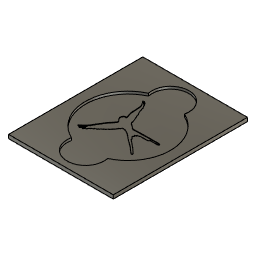
Wingspan - Food Token Lid (Autodesk Fusion 360 design; units mm, degrees)
Autodesk Fusion 360 part; units mm, degrees
(part 1 of 2)
sketch "Skizze1" plane through (0, 0, 0) normal (0, 0, 1) x (1, 0, 0)
  line L0 (0, 0) -> (85, 0)
  line L1 (85, 0) -> (85, 109)
  line L2 (85, 109) -> (0, 109)
  line L3 (0, 109) -> (0, 0)
  line L4 (0, 0) -> (7, 0)
  line L5 (7, 0) -> (7, 7)
  line L6 (7, 7) -> (0, 7)
  line L7 (0, 7) -> (0, 0)
  line L8 (85, 0) -> (78, 0)
  line L9 (78, 0) -> (78, 7)
  line L10 (78, 7) -> (85, 7)
  line L11 (85, 7) -> (85, 0)
  line L12 (85, 109) -> (78, 109)
  line L13 (78, 109) -> (78, 102)
  line L14 (78, 102) -> (85, 102)
  line L15 (85, 102) -> (85, 109)
  line L16 (0, 109) -> (7, 109)
  line L17 (7, 109) -> (7, 102)
  line L18 (7, 102) -> (0, 102)
  line L19 (0, 102) -> (0, 109)
  circle A0 centre (3.5, 3.5) radius 2.65
  circle A1 centre (81.5, 3.5) radius 2.65
  circle A2 centre (81.5, 105.5) radius 2.65
  circle A3 centre (3.5, 105.5) radius 2.65
  dimension "d1" = 85
  dimension "d2" = 109
  dimension "d3" = 7
  dimension "d4" = 7
  dimension "d5" = 7
  dimension "d6" = 7
  dimension "d7" = 7
  dimension "d8" = 7
  dimension "d9" = 7
  dimension "d10" = 7
  dimension "d11" = 5.3
  dimension "d12" = 5.3
  dimension "d13" = 5.3
  dimension "d14" = 5.3
  dimension "d15" = 3.5
  dimension "d16" = 3.5
  dimension "d17" = 3.5
  dimension "d18" = 3.5
  dimension "d19" = 3.5
  dimension "d20" = 3.5
  dimension "d21" = 3.5
  dimension "d22" = 3.5
  constraint horizontal L0
  constraint vertical L1
  constraint horizontal L2
  constraint vertical L3
  constraint coincident L0.start L3.end
  constraint horizontal L4
  constraint vertical L5
  constraint horizontal L6
  constraint vertical L7
  constraint horizontal L8
  constraint vertical L9
  constraint horizontal L10
  constraint vertical L11
  constraint horizontal L12
  constraint vertical L13
  constraint horizontal L14
  constraint vertical L15
  constraint horizontal L16
  constraint vertical L17
  constraint horizontal L18
  constraint vertical L19
  measures "d1" distance of L0.start L0.end
  measures "d2" distance of L0.start L2.end
  measures "d3" distance of L0.start L4.end
  measures "d4" distance of L0.start L6.end
  measures "d5" distance of L0.end L8.end
  measures "d6" distance of L0.end L10.end
  measures "d7" distance of L1.end L12.end
  measures "d8" distance of L1.end L14.end
  measures "d9" distance of L2.end L16.end
  measures "d10" distance of L2.end L18.end
  measures "d11" diameter of A0
  measures "d12" diameter of A1
  measures "d13" diameter of A2
  measures "d14" diameter of A3
  measures "d15" distance of L19 A3.centre
  measures "d16" distance of L16 A3.centre
  measures "d17" distance of L2 A2.centre
  measures "d18" distance of L1 A2.centre
  measures "d19" distance of L1 A1.centre
  measures "d20" distance of L0 A1.centre
  measures "d21" distance of L0 A0.centre
  measures "d22" distance of L5 A0.centre
extrude "Extrusion3" add sketch "Skizze1" along normal blind 3 contours L0 L3 L4 L5 L6 L7 | L0 L1 L2 L3 L5 L6 L9 L10 L13 L14 L17 L18 | L0 L1 L8 L9 L10 L11 | L2 L3 L16 L17 L18 L19 | L1 L2 L12 L13 L14 L15 | A0 | A1 | A2 | A3
extrude "Extrusion4" cut sketch "Skizze1" along normal blind 1.2 contours A0 | A1 | A2 | A3
sketch "Skizze3" plane through (0, 0, 3) normal (0, 0, 1) x (-1, 0, 0)
  line L0 (0, -109) -> (0, 0)
  line L1 (0, 0) -> (-85, 0)
  line L2 (-85, 0) -> (-85, -109)
  line L3 (-85, -109) -> (0, -109)
  circle A0 centre (-42.5, -54.5) radius 34.5
  circle A1 centre (-42.5, -89) radius 15
  circle A2 centre (-42.5, -20) radius 15
  dimension "d39" = 69
  dimension "d40" = 42.5
  dimension "d50" = 30
  dimension "d51" = 30
  dimension "d52" = 20
  dimension "d53" = 20
  constraint coincident A0 A1.centre
  constraint coincident A0 A2.centre
  measures "d39" diameter of A0
  measures "d40" distance of L2 A0.centre
  measures "d50" diameter of A1
  measures "d51" diameter of A2
  measures "d52" distance of L1 A2.centre
  measures "d53" distance of L3 A1.centre
extrude "Extrusion7" cut sketch "Skizze3" against normal blind 2 contours A0 A1 A2 | A0 A2 | A0 A2 | A0 A1 | A0 A1
sketch "Skizze5" plane through (0, 0, 1) normal (0, 0, 1) x (-1, 0, 0)
  arc A0 (-27.8587, -23.2609) -> (-57.1413, -23.2609) centre (-42.5, -20) ccw
  arc A1 (-57.1413, -23.2609) -> (-57.1413, -85.7391) centre (-42.5, -54.5) ccw
  arc A2 (-57.1413, -85.7391) -> (-27.8587, -85.7391) centre (-42.5, -89) ccw
  arc A3 (-27.8587, -85.7391) -> (-27.8587, -23.2609) centre (-42.5, -54.5) ccw
  spline S0 degree 3 poles (-66.4769, -55.696) (-66.34, -55.5333) (-66.0829, -55.391) (-65.7535, -55.2957) knots 0 0 0 0 1 1 1 1
  spline S1 degree 3 poles (-65.7535, -55.2957) (-65.527, -55.2301) (-64.4525, -55.1908) (-60.9377, -55.1195) knots 0 0 0 0 1 1 1 1
  line L0 (-60.9377, -55.1195) -> (-59.6311, -55.0929)
  line L1 (-59.6311, -55.0929) -> (-59.5794, -54.9682)
  spline S2 degree 3 poles (-59.5794, -54.9682) (-59.551, -54.8996) (-59.4198, -54.7368) (-59.2878, -54.6065) knots 0 0 0 0 1 1 1 1
  spline S3 degree 3 poles (-59.2878, -54.6065) (-59.1032, -54.4242) (-58.9697, -54.341) (-58.7092, -54.2459) knots 0 0 0 0 1 1 1 1
  line L2 (-58.7092, -54.2459) -> (-58.3706, -54.1223)
  line L3 (-58.3706, -54.1223) -> (-56.297, -54.1159)
  spline S4 degree 3 poles (-56.297, -54.1159) (-55.1565, -54.1124) (-53.92, -54.1227) (-53.5492, -54.1387) knots 0 0 0 0 1 1 1 1
  line L4 (-53.5492, -54.1387) -> (-52.875, -54.1678)
  line L5 (-52.875, -54.1678) -> (-52.7061, -53.9931)
  spline S5 degree 3 poles (-52.7061, -53.9931) (-52.3675, -53.6427) (-52.283, -53.6204) (-51.3104, -53.6252) knots 0 0 0 0 1 1 1 1
  line L6 (-51.3104, -53.6252) -> (-50.4482, -53.6294)
  line L7 (-50.4482, -53.6294) -> (-50.6724, -53.5227)
  spline S6 degree 3 poles (-50.6724, -53.5227) (-51.098, -53.3202) (-51.2581, -53.0214) (-51.0466, -52.8244) knots 0 0 0 0 1 1 1 1
  spline S7 degree 3 poles (-51.0466, -52.8244) (-50.8983, -52.6862) (-50.6376, -52.6297) (-50.0763, -52.6141) knots 0 0 0 0 1 1 1 1
  spline S8 degree 3 poles (-50.0763, -52.6141) (-49.8005, -52.6065) (-49.5647, -52.5989) (-49.5522, -52.5973) knots 0 0 0 0 1 1 1 1
  spline S9 degree 3 poles (-49.5522, -52.5973) (-49.5396, -52.5958) (-49.6513, -52.5267) (-49.8002, -52.4438) knots 0 0 0 0 1 1 1 1
  spline S10 degree 3 poles (-49.8002, -52.4438) (-50.1699, -52.2381) (-50.2586, -52.1091) (-50.2586, -51.7767) knots 0 0 0 0 1 1 1 1
  spline S11 degree 3 poles (-50.2586, -51.7767) (-50.2586, -51.5758) (-50.2364, -51.4865) (-50.1674, -51.4091) knots 0 0 0 0 1 1 1 1
  spline S12 degree 3 poles (-50.1674, -51.4091) (-50.0289, -51.2538) (-49.7965, -51.172) (-49.592, -51.2065) knots 0 0 0 0 1 1 1 1
  spline S13 degree 3 poles (-49.592, -51.2065) (-49.3888, -51.2409) (-49.3721, -51.2026) (-49.5262, -51.0565) knots 0 0 0 0 1 1 1 1
  spline S14 degree 3 poles (-49.5262, -51.0565) (-49.5863, -50.9995) (-49.662, -50.8491) (-49.6945, -50.7222) knots 0 0 0 0 1 1 1 1
  spline S15 degree 3 poles (-49.6945, -50.7222) (-49.7368, -50.5571) (-49.7967, -50.4568) (-49.9045, -50.3699) knots 0 0 0 0 1 1 1 1
  spline S16 degree 3 poles (-49.9045, -50.3699) (-50.9398, -49.5366) (-51.2613, -49.1022) (-51.2611, -48.537) knots 0 0 0 0 1 1 1 1
  line L8 (-51.2611, -48.537) -> (-51.261, -48.2382)
  line L9 (-51.261, -48.2382) -> (-51.6839, -47.9217)
  spline S17 degree 3 poles (-51.6839, -47.9217) (-52.6699, -47.184) (-53.8348, -46.2825) (-54.2425, -45.9418) knots 0 0 0 0 1 1 1 1
  spline S18 degree 3 poles (-54.2425, -45.9418) (-54.4075, -45.8039) (-54.6394, -45.6132) (-54.7578, -45.5181) knots 0 0 0 0 1 1 1 1
  spline S19 degree 3 poles (-54.7578, -45.5181) (-54.8763, -45.423) (-54.9993, -45.3205) (-55.0313, -45.2903) knots 0 0 0 0 1 1 1 1
  spline S20 degree 3 poles (-55.0313, -45.2903) (-55.0633, -45.2601) (-55.2433, -45.1022) (-55.4312, -44.9393) knots 0 0 0 0 1 1 1 1
  spline S21 degree 3 poles (-55.4312, -44.9393) (-55.6192, -44.7764) (-55.7832, -44.632) (-55.7957, -44.6185) knots 0 0 0 0 1 1 1 1
  spline S22 degree 3 poles (-55.7957, -44.6185) (-55.8083, -44.605) (-56.0339, -44.4246) (-56.297, -44.2177) knots 0 0 0 0 1 1 1 1
  spline S23 degree 3 poles (-56.297, -44.2177) (-57.2107, -43.4994) (-57.9229, -42.9318) (-58.0098, -42.8527) knots 0 0 0 0 1 1 1 1
  spline S24 degree 3 poles (-58.0098, -42.8527) (-58.0579, -42.8089) (-58.156, -42.7275) (-58.2279, -42.6719) knots 0 0 0 0 1 1 1 1
  spline S25 degree 3 poles (-58.2279, -42.6719) (-58.4581, -42.4936) (-58.8082, -42.168) (-59.5801, -41.4142) knots 0 0 0 0 1 1 1 1
  spline S26 degree 3 poles (-59.5801, -41.4142) (-59.9946, -41.0094) (-60.4764, -40.5551) (-60.6506, -40.4047) knots 0 0 0 0 1 1 1 1
  spline S27 degree 3 poles (-60.6506, -40.4047) (-61.2019, -39.9288) (-61.5559, -39.5916) (-61.7517, -39.3554) knots 0 0 0 0 1 1 1 1
  spline S28 degree 3 poles (-61.7517, -39.3554) (-62.1736, -38.8466) (-62.3005, -38.3445) (-62.0559, -38.1521) knots 0 0 0 0 1 1 1 1
  spline S29 degree 3 poles (-62.0559, -38.1521) (-61.9898, -38.1002) (-61.8911, -38.0577) (-61.8365, -38.0577) knots 0 0 0 0 1 1 1 1
  spline S30 degree 3 poles (-61.8365, -38.0577) (-61.5957, -38.0577) (-61.0744, -38.3909) (-60.2553, -39.0684) knots 0 0 0 0 1 1 1 1
  spline S31 degree 3 poles (-60.2553, -39.0684) (-59.6798, -39.5445) (-57.8513, -41.1473) (-57.4333, -41.5422) knots 0 0 0 0 1 1 1 1
  spline S32 degree 3 poles (-57.4333, -41.5422) (-56.8243, -42.1176) (-56.0099, -42.7891) (-55.4142, -43.2072) knots 0 0 0 0 1 1 1 1
  spline S33 degree 3 poles (-55.4142, -43.2072) (-55.3608, -43.2446) (-55.1224, -43.425) (-54.8842, -43.6081) knots 0 0 0 0 1 1 1 1
  spline S34 degree 3 poles (-54.8842, -43.6081) (-54.6461, -43.7911) (-54.2975, -44.0573) (-54.1095, -44.1995) knots 0 0 0 0 1 1 1 1
  spline S35 degree 3 poles (-54.1095, -44.1995) (-53.9215, -44.3418) (-53.7574, -44.47) (-53.7449, -44.4844) knots 0 0 0 0 1 1 1 1
  spline S36 degree 3 poles (-53.7449, -44.4844) (-53.6626, -44.579) (-52.9747, -45.0648) (-52.1726, -45.5948) knots 0 0 0 0 1 1 1 1
  spline S37 degree 3 poles (-52.1726, -45.5948) (-51.947, -45.7439) (-51.5599, -46.0213) (-51.3124, -46.2115) knots 0 0 0 0 1 1 1 1
  spline S38 degree 3 poles (-51.3124, -46.2115) (-51.0649, -46.4016) (-50.6119, -46.7417) (-50.3058, -46.9672) knots 0 0 0 0 1 1 1 1
  spline S39 degree 3 poles (-50.3058, -46.9672) (-49.9997, -47.1928) (-49.6491, -47.4594) (-49.5267, -47.5597) knots 0 0 0 0 1 1 1 1
  spline S40 degree 3 poles (-49.5267, -47.5597) (-49.4043, -47.66) (-49.2625, -47.7758) (-49.2117, -47.8172) knots 0 0 0 0 1 1 1 1
  spline S41 degree 3 poles (-49.2117, -47.8172) (-48.9391, -48.0387) (-48.6357, -48.303) (-48.4128, -48.5129) knots 0 0 0 0 1 1 1 1
  spline S42 degree 3 poles (-48.4128, -48.5129) (-47.9347, -48.9631) (-47.2927, -49.4869) (-46.5933, -49.9973) knots 0 0 0 0 1 1 1 1
  spline S43 degree 3 poles (-46.5933, -49.9973) (-46.2067, -50.2794) (-45.8395, -50.5574) (-45.7774, -50.615) knots 0 0 0 0 1 1 1 1
  spline S44 degree 3 poles (-45.7774, -50.615) (-45.7153, -50.6726) (-45.552, -50.7628) (-45.4146, -50.8154) knots 0 0 0 0 1 1 1 1
  spline S45 degree 3 poles (-45.4146, -50.8154) (-45.2771, -50.868) (-45.034, -51.0024) (-44.8742, -51.114) knots 0 0 0 0 1 1 1 1
  spline S46 degree 3 poles (-44.8742, -51.114) (-44.7145, -51.2257) (-44.4968, -51.3657) (-44.3905, -51.4251) knots 0 0 0 0 1 1 1 1
  spline S47 degree 3 poles (-44.3905, -51.4251) (-44.2843, -51.4846) (-44.0127, -51.6369) (-43.7871, -51.7636) knots 0 0 0 0 1 1 1 1
  spline S48 degree 3 poles (-43.7871, -51.7636) (-43.2146, -52.0851) (-42.9986, -52.1776) (-42.3972, -52.3586) knots 0 0 0 0 1 1 1 1
  spline S49 degree 3 poles (-42.3972, -52.3586) (-42.3094, -52.385) (-42.0736, -52.4366) (-41.8731, -52.4733) knots 0 0 0 0 1 1 1 1
  spline S50 degree 3 poles (-41.8731, -52.4733) (-40.6244, -52.7018) (-40.1267, -52.7538) (-40.0297, -52.666) knots 0 0 0 0 1 1 1 1
  spline S51 degree 3 poles (-40.0297, -52.666) (-39.9907, -52.6308) (-39.9025, -52.5805) (-39.8336, -52.5543) knots 0 0 0 0 1 1 1 1
  spline S52 degree 3 poles (-39.8336, -52.5543) (-39.7276, -52.514) (-39.7083, -52.4802) (-39.7079, -52.3346) knots 0 0 0 0 1 1 1 1
  spline S53 degree 3 poles (-39.7079, -52.3346) (-39.7074, -52.1249) (-39.5052, -51.7553) (-39.2857, -51.5625) knots 0 0 0 0 1 1 1 1
  spline S54 degree 3 poles (-39.2857, -51.5625) (-39.1997, -51.487) (-38.9728, -51.3245) (-38.7815, -51.2015) knots 0 0 0 0 1 1 1 1
  spline S55 degree 3 poles (-38.7815, -51.2015) (-38.4753, -51.0044) (-38.4336, -50.9613) (-38.433, -50.8403) knots 0 0 0 0 1 1 1 1
  spline S56 degree 3 poles (-38.433, -50.8403) (-38.4319, -50.6375) (-38.2757, -50.3745) (-37.9723, -50.065) knots 0 0 0 0 1 1 1 1
  spline S57 degree 3 poles (-37.9723, -50.065) (-37.7651, -49.8536) (-37.7031, -49.759) (-37.7031, -49.6542) knots 0 0 0 0 1 1 1 1
  spline S58 degree 3 poles (-37.7031, -49.6542) (-37.7031, -49.3952) (-37.486, -49.0956) (-36.7303, -48.3117) knots 0 0 0 0 1 1 1 1
  spline S59 degree 3 poles (-36.7303, -48.3117) (-36.605, -48.1817) (-36.5214, -48.0471) (-36.5021, -47.9442) knots 0 0 0 0 1 1 1 1
  spline S60 degree 3 poles (-36.5021, -47.9442) (-36.4668, -47.7556) (-36.3035, -47.5861) (-35.8816, -47.2996) knots 0 0 0 0 1 1 1 1
  spline S61 degree 3 poles (-35.8816, -47.2996) (-35.6517, -47.1435) (-35.5802, -47.0676) (-35.5572, -46.9547) knots 0 0 0 0 1 1 1 1
  spline S62 degree 3 poles (-35.5572, -46.9547) (-35.5232, -46.7888) (-35.4056, -46.595) (-35.2684, -46.4787) knots 0 0 0 0 1 1 1 1
  spline S63 degree 3 poles (-35.2684, -46.4787) (-35.1092, -46.3439) (-34.6422, -46.1241) (-34.5148, -46.1241) knots 0 0 0 0 1 1 1 1
  spline S64 degree 3 poles (-34.5148, -46.1241) (-34.3507, -46.1241) (-34.2851, -46.0455) (-34.2851, -45.8486) knots 0 0 0 0 1 1 1 1
  spline S65 degree 3 poles (-34.2851, -45.8486) (-34.2851, -45.6239) (-34.1771, -45.4147) (-33.9272, -45.1554) knots 0 0 0 0 1 1 1 1
  spline S66 degree 3 poles (-33.9272, -45.1554) (-33.7648, -44.9869) (-33.6355, -44.9073) (-33.3475, -44.7986) knots 0 0 0 0 1 1 1 1
  line L10 (-33.3475, -44.7986) -> (-32.9769, -44.6588)
  line L11 (-32.9769, -44.6588) -> (-32.845, -44.3828)
  spline S67 degree 3 poles (-32.845, -44.3828) (-32.7703, -44.2264) (-32.631, -44.0346) (-32.5238, -43.9402) knots 0 0 0 0 1 1 1 1
  spline S68 degree 3 poles (-32.5238, -43.9402) (-32.2976, -43.7411) (-31.8763, -43.5265) (-31.7117, -43.5265) knots 0 0 0 0 1 1 1 1
  spline S69 degree 3 poles (-31.7117, -43.5265) (-31.6466, -43.5265) (-31.5858, -43.5008) (-31.5764, -43.4695) knots 0 0 0 0 1 1 1 1
  spline S70 degree 3 poles (-31.5764, -43.4695) (-31.4482, -43.041) (-31.3897, -42.8961) (-31.2943, -42.771) knots 0 0 0 0 1 1 1 1
  spline S71 degree 3 poles (-31.2943, -42.771) (-31.1591, -42.5937) (-31.0965, -42.563) (-30.7991, -42.5279) knots 0 0 0 0 1 1 1 1
  spline S72 degree 3 poles (-30.7991, -42.5279) (-30.6026, -42.5047) (-30.5683, -42.4855) (-30.5484, -42.3871) knots 0 0 0 0 1 1 1 1
  spline S73 degree 3 poles (-30.5484, -42.3871) (-30.5357, -42.3245) (-30.468, -42.1707) (-30.3978, -42.0453) knots 0 0 0 0 1 1 1 1
  spline S74 degree 3 poles (-30.3978, -42.0453) (-30.1637, -41.6269) (-29.6643, -41.3954) (-29.1645, -41.4736) knots 0 0 0 0 1 1 1 1
  line L12 (-29.1645, -41.4736) -> (-28.943, -41.5083)
  line L13 (-28.943, -41.5083) -> (-28.8747, -41.3439)
  spline S75 degree 3 poles (-28.8747, -41.3439) (-28.5136, -40.4738) (-28.2322, -40.1996) (-27.7003, -40.1996) knots 0 0 0 0 1 1 1 1
  spline S76 degree 3 poles (-27.7003, -40.1996) (-27.5176, -40.1996) (-27.4862, -40.1846) (-27.4379, -40.0743) knots 0 0 0 0 1 1 1 1
  spline S77 degree 3 poles (-27.4379, -40.0743) (-27.3216, -39.8085) (-26.9953, -39.3413) (-26.8574, -39.2431) knots 0 0 0 0 1 1 1 1
  spline S78 degree 3 poles (-26.8574, -39.2431) (-26.7338, -39.1551) (-26.6213, -39.1237) (-26.3759, -39.1088) knots 0 0 0 0 1 1 1 1
  spline S79 degree 3 poles (-26.3759, -39.1088) (-26.3496, -39.1072) (-26.3014, -39.029) (-26.2687, -38.935) knots 0 0 0 0 1 1 1 1
  spline S80 degree 3 poles (-26.2687, -38.935) (-26.0867, -38.4114) (-25.7297, -37.7861) (-25.5326, -37.6458) knots 0 0 0 0 1 1 1 1
  spline S81 degree 3 poles (-25.5326, -37.6458) (-25.3618, -37.5242) (-25.2466, -37.5595) (-25.1499, -37.7631) knots 0 0 0 0 1 1 1 1
  spline S82 degree 3 poles (-25.1499, -37.7631) (-25.1087, -37.8499) (-25.0606, -37.9209) (-25.043, -37.9208) knots 0 0 0 0 1 1 1 1
  spline S83 degree 3 poles (-25.043, -37.9208) (-25.0254, -37.9207) (-24.9723, -37.8266) (-24.925, -37.7116) knots 0 0 0 0 1 1 1 1
  spline S84 degree 3 poles (-24.925, -37.7116) (-24.6067, -36.9378) (-23.588, -35.957) (-23.457, -36.2982) knots 0 0 0 0 1 1 1 1
  spline S85 degree 3 poles (-23.457, -36.2982) (-23.4357, -36.3538) (-23.5936, -36.8575) (-23.7586, -37.2601) knots 0 0 0 0 1 1 1 1
  spline S86 degree 3 poles (-23.7586, -37.2601) (-23.8232, -37.4177) (-23.8414, -37.4655) (-24.0021, -37.8982) knots 0 0 0 0 1 1 1 1
  spline S87 degree 3 poles (-24.0021, -37.8982) (-24.1251, -38.2292) (-24.1962, -38.5134) (-24.1561, -38.5134) knots 0 0 0 0 1 1 1 1
  spline S88 degree 3 poles (-24.1561, -38.5134) (-24.1433, -38.5134) (-24.0038, -38.334) (-23.846, -38.1146) knots 0 0 0 0 1 1 1 1
  spline S89 degree 3 poles (-23.846, -38.1146) (-23.5032, -37.6383) (-22.5753, -36.5191) (-22.2944, -36.2433) knots 0 0 0 0 1 1 1 1
  spline S90 degree 3 poles (-22.2944, -36.2433) (-21.9373, -35.8927) (-21.479, -35.6325) (-21.479, -35.7804) knots 0 0 0 0 1 1 1 1
  spline S91 degree 3 poles (-21.479, -35.7804) (-21.479, -35.8063) (-21.679, -36.0602) (-21.9234, -36.3448) knots 0 0 0 0 1 1 1 1
  spline S92 degree 3 poles (-21.9234, -36.3448) (-22.4445, -36.9516) (-22.5938, -37.14) (-22.7745, -37.4189) knots 0 0 0 0 1 1 1 1
  spline S93 degree 3 poles (-22.7745, -37.4189) (-23.0018, -37.7697) (-23.2586, -38.253) (-23.2318, -38.2797) knots 0 0 0 0 1 1 1 1
  spline S94 degree 3 poles (-23.2318, -38.2797) (-23.2178, -38.2937) (-22.8638, -37.9588) (-22.4452, -37.5353) knots 0 0 0 0 1 1 1 1
  spline S95 degree 3 poles (-22.4452, -37.5353) (-21.8538, -36.937) (-21.579, -36.6961) (-21.2126, -36.4545) knots 0 0 0 0 1 1 1 1
  spline S96 degree 3 poles (-21.2126, -36.4545) (-20.948, -36.28) (-20.6914, -36.1436) (-20.6278, -36.1436) knots 0 0 0 0 1 1 1 1
  spline S97 degree 3 poles (-20.6278, -36.1436) (-20.4556, -36.1436) (-20.5179, -36.2337) (-20.8387, -36.4486) knots 0 0 0 0 1 1 1 1
  spline S98 degree 3 poles (-20.8387, -36.4486) (-21.1871, -36.6821) (-21.5614, -37.004) (-22.0473, -37.4881) knots 0 0 0 0 1 1 1 1
  spline S99 degree 3 poles (-22.0473, -37.4881) (-22.7212, -38.1595) (-23.0746, -38.62) (-23.6485, -39.5745) knots 0 0 0 0 1 1 1 1
  spline S100 degree 3 poles (-23.6485, -39.5745) (-23.9868, -40.137) (-24.0053, -40.2286) (-23.7285, -39.97) knots 0 0 0 0 1 1 1 1
  spline S101 degree 3 poles (-23.7285, -39.97) (-23.5024, -39.7589) (-23.346, -39.6291) (-22.6639, -39.0863) knots 0 0 0 0 1 1 1 1
  spline S102 degree 3 poles (-22.6639, -39.0863) (-22.4509, -38.9168) (-22.1433, -38.6518) (-21.9803, -38.4974) knots 0 0 0 0 1 1 1 1
  spline S103 degree 3 poles (-21.9803, -38.4974) (-21.3863, -37.9344) (-20.9782, -37.5964) (-20.5158, -37.2843) knots 0 0 0 0 1 1 1 1
  spline S104 degree 3 poles (-20.5158, -37.2843) (-20.256, -37.109) (-19.9438, -36.8934) (-19.822, -36.8052) knots 0 0 0 0 1 1 1 1
  spline S105 degree 3 poles (-19.822, -36.8052) (-19.6003, -36.6447) (-19.458, -36.6054) (-19.4057, -36.6901) knots 0 0 0 0 1 1 1 1
  spline S106 degree 3 poles (-19.4057, -36.6901) (-19.3728, -36.7433) (-19.4722, -36.8384) (-19.9779, -37.2374) knots 0 0 0 0 1 1 1 1
  spline S107 degree 3 poles (-19.9779, -37.2374) (-20.988, -38.0342) (-21.6759, -38.6504) (-22.5637, -39.5537) knots 0 0 0 0 1 1 1 1
  spline S108 degree 3 poles (-22.5637, -39.5537) (-23.0976, -40.0969) (-23.6206, -40.6605) (-23.7258, -40.8061) knots 0 0 0 0 1 1 1 1
  spline S109 degree 3 poles (-23.7258, -40.8061) (-23.8311, -40.9516) (-24.0012, -41.1807) (-24.1038, -41.3152) knots 0 0 0 0 1 1 1 1
  spline S110 degree 3 poles (-24.1038, -41.3152) (-24.5569, -41.9085) (-25.3728, -43.1972) (-25.706, -43.8455) knots 0 0 0 0 1 1 1 1
  spline S111 degree 3 poles (-25.706, -43.8455) (-26.1808, -44.7695) (-26.3303, -45.0267) (-26.7764, -45.6872) knots 0 0 0 0 1 1 1 1
  spline S112 degree 3 poles (-26.7764, -45.6872) (-27.6231, -46.9408) (-28.2239, -47.8712) (-28.2239, -47.9288) knots 0 0 0 0 1 1 1 1
  spline S113 degree 3 poles (-28.2239, -47.9288) (-28.2239, -47.9399) (-28.272, -48.0254) (-28.3309, -48.1189) knots 0 0 0 0 1 1 1 1
  spline S114 degree 3 poles (-28.3309, -48.1189) (-28.3897, -48.2124) (-28.51, -48.4222) (-28.5981, -48.5851) knots 0 0 0 0 1 1 1 1
  spline S115 degree 3 poles (-28.5981, -48.5851) (-28.6863, -48.748) (-28.8057, -48.9634) (-28.8636, -49.0636) knots 0 0 0 0 1 1 1 1
  spline S116 degree 3 poles (-28.8636, -49.0636) (-28.9215, -49.1639) (-29.0219, -49.3382) (-29.0867, -49.451) knots 0 0 0 0 1 1 1 1
  spline S117 degree 3 poles (-29.0867, -49.451) (-29.1515, -49.5638) (-29.2761, -49.7575) (-29.3636, -49.8815) knots 0 0 0 0 1 1 1 1
  spline S118 degree 3 poles (-29.3636, -49.8815) (-29.6443, -50.2791) (-31.007, -51.9697) (-31.865, -52.9847) knots 0 0 0 0 1 1 1 1
  spline S119 degree 3 poles (-31.865, -52.9847) (-32.0366, -53.1877) (-32.8129, -54.2308) (-32.9999, -54.5096) knots 0 0 0 0 1 1 1 1
  spline S120 degree 3 poles (-32.9999, -54.5096) (-33.4602, -55.196) (-33.5128, -55.3056) (-33.5059, -55.5654) knots 0 0 0 0 1 1 1 1
  spline S121 degree 3 poles (-33.5059, -55.5654) (-33.4939, -56.0167) (-33.2865, -56.3551) (-32.7659, -56.7729) knots 0 0 0 0 1 1 1 1
  spline S122 degree 3 poles (-32.7659, -56.7729) (-31.8731, -57.4895) (-31.4629, -58.0581) (-31.2493, -58.8755) knots 0 0 0 0 1 1 1 1
  spline S123 degree 3 poles (-31.2493, -58.8755) (-31.1724, -59.1695) (-31.1648, -60.1497) (-31.238, -60.3295) knots 0 0 0 0 1 1 1 1
  spline S124 degree 3 poles (-31.238, -60.3295) (-31.5742, -61.1551) (-31.915, -61.6094) (-32.3837, -61.8568) knots 0 0 0 0 1 1 1 1
  spline S125 degree 3 poles (-32.3837, -61.8568) (-32.6571, -62.0011) (-33.3043, -62.0003) (-33.5987, -61.8554) knots 0 0 0 0 1 1 1 1
  spline S126 degree 3 poles (-33.5987, -61.8554) (-34.0207, -61.6476) (-34.0797, -61.7272) (-33.9054, -62.2693) knots 0 0 0 0 1 1 1 1
  spline S127 degree 3 poles (-33.9054, -62.2693) (-33.831, -62.5007) (-33.7563, -62.7208) (-33.7395, -62.7584) knots 0 0 0 0 1 1 1 1
  spline S128 degree 3 poles (-33.7395, -62.7584) (-33.6155, -63.0353) (-32.7433, -65.8249) (-32.6423, -66.2675) knots 0 0 0 0 1 1 1 1
  spline S129 degree 3 poles (-32.6423, -66.2675) (-32.6108, -66.4054) (-32.5574, -66.6062) (-32.5236, -66.7137) knots 0 0 0 0 1 1 1 1
  spline S130 degree 3 poles (-32.5236, -66.7137) (-32.357, -67.2428) (-32.3173, -67.6943) (-32.3001, -69.2526) knots 0 0 0 0 1 1 1 1
  spline S131 degree 3 poles (-32.3001, -69.2526) (-32.2908, -70.1048) (-32.2639, -70.9456) (-32.2404, -71.1211) knots 0 0 0 0 1 1 1 1
  spline S132 degree 3 poles (-32.2404, -71.1211) (-32.1632, -71.6977) (-32.1063, -72.2947) (-32.0557, -73.0579) knots 0 0 0 0 1 1 1 1
  spline S133 degree 3 poles (-32.0557, -73.0579) (-31.9862, -74.1079) (-31.8116, -75.4244) (-31.6841, -75.8607) knots 0 0 0 0 1 1 1 1
  spline S134 degree 3 poles (-31.6841, -75.8607) (-31.4966, -76.5023) (-31.3516, -76.7732) (-30.7569, -77.5925) knots 0 0 0 0 1 1 1 1
  spline S135 degree 3 poles (-30.7569, -77.5925) (-29.8366, -78.8604) (-29.6535, -79.1189) (-29.4185, -79.4825) knots 0 0 0 0 1 1 1 1
  spline S136 degree 3 poles (-29.4185, -79.4825) (-28.9782, -80.1639) (-28.9489, -80.2297) (-29.0663, -80.2748) knots 0 0 0 0 1 1 1 1
  spline S137 degree 3 poles (-29.0663, -80.2748) (-29.1292, -80.2989) (-29.4694, -80.0351) (-29.9784, -79.5675) knots 0 0 0 0 1 1 1 1
  spline S138 degree 3 poles (-29.9784, -79.5675) (-30.0787, -79.4754) (-30.2149, -79.3577) (-30.281, -79.3059) knots 0 0 0 0 1 1 1 1
  spline S139 degree 3 poles (-30.281, -79.3059) (-30.3471, -79.2541) (-30.5108, -79.0767) (-30.6446, -78.9118) knots 0 0 0 0 1 1 1 1
  spline S140 degree 3 poles (-30.6446, -78.9118) (-30.7784, -78.7468) (-30.8953, -78.6339) (-30.9042, -78.6608) knots 0 0 0 0 1 1 1 1
  spline S141 degree 3 poles (-30.9042, -78.6608) (-30.947, -78.7891) (-30.1803, -79.9438) (-29.8888, -80.1902) knots 0 0 0 0 1 1 1 1
  spline S142 degree 3 poles (-29.8888, -80.1902) (-29.8591, -80.2152) (-29.7982, -80.2921) (-29.7533, -80.3611) knots 0 0 0 0 1 1 1 1
  spline S143 degree 3 poles (-29.7533, -80.3611) (-29.6732, -80.4841) (-29.6735, -80.4864) (-29.7691, -80.4864) knots 0 0 0 0 1 1 1 1
  spline S144 degree 3 poles (-29.7691, -80.4864) (-29.8519, -80.4864) (-30.0572, -80.3286) (-30.3633, -80.0298) knots 0 0 0 0 1 1 1 1
  spline S145 degree 3 poles (-30.3633, -80.0298) (-30.7613, -79.6411) (-31.2149, -78.9699) (-31.4855, -78.369) knots 0 0 0 0 1 1 1 1
  spline S146 degree 3 poles (-31.4855, -78.369) (-31.6468, -78.0109) (-31.7338, -77.8939) (-31.7325, -78.0368) knots 0 0 0 0 1 1 1 1
  spline S147 degree 3 poles (-31.7325, -78.0368) (-31.7316, -78.1411) (-31.4114, -79.0011) (-31.2979, -79.2041) knots 0 0 0 0 1 1 1 1
  spline S148 degree 3 poles (-31.2979, -79.2041) (-31.1648, -79.4424) (-31.157, -79.5293) (-31.269, -79.5293) knots 0 0 0 0 1 1 1 1
  spline S149 degree 3 poles (-31.269, -79.5293) (-31.4614, -79.5293) (-32.1902, -78.2413) (-32.4424, -77.4558) knots 0 0 0 0 1 1 1 1
  spline S150 degree 3 poles (-32.4424, -77.4558) (-32.5482, -77.126) (-32.61, -77.0823) (-32.6358, -77.319) knots 0 0 0 0 1 1 1 1
  spline S151 degree 3 poles (-32.6358, -77.319) (-32.656, -77.5053) (-32.7468, -77.5978) (-32.8212, -77.5081) knots 0 0 0 0 1 1 1 1
  spline S152 degree 3 poles (-32.8212, -77.5081) (-32.8699, -77.4494) (-33.2525, -76.4156) (-33.3129, -76.1797) knots 0 0 0 0 1 1 1 1
  spline S153 degree 3 poles (-33.3129, -76.1797) (-33.3583, -76.0024) (-33.4868, -75.7915) (-33.5646, -75.7668) knots 0 0 0 0 1 1 1 1
  spline S154 degree 3 poles (-33.5646, -75.7668) (-33.6451, -75.7412) (-33.9953, -75.2362) (-34.0955, -75.0011) knots 0 0 0 0 1 1 1 1
  spline S155 degree 3 poles (-34.0955, -75.0011) (-34.1261, -74.9293) (-34.164, -74.6422) (-34.1796, -74.363) knots 0 0 0 0 1 1 1 1
  spline S156 degree 3 poles (-34.1796, -74.363) (-34.2081, -73.8564) (-34.2085, -73.8551) (-34.3812, -73.6578) knots 0 0 0 0 1 1 1 1
  spline S157 degree 3 poles (-34.3812, -73.6578) (-34.6559, -73.344) (-34.742, -73.12) (-34.7815, -72.6162) knots 0 0 0 0 1 1 1 1
  spline S158 degree 3 poles (-34.7815, -72.6162) (-34.8145, -72.1951) (-34.8288, -72.1481) (-35.0294, -71.8037) knots 0 0 0 0 1 1 1 1
  spline S159 degree 3 poles (-35.0294, -71.8037) (-35.1724, -71.5582) (-35.2774, -71.2996) (-35.3489, -71.0169) knots 0 0 0 0 1 1 1 1
  spline S160 degree 3 poles (-35.3489, -71.0169) (-35.4089, -70.7795) (-35.4962, -70.5512) (-35.5489, -70.4938) knots 0 0 0 0 1 1 1 1
  spline S161 degree 3 poles (-35.5489, -70.4938) (-35.7137, -70.3142) (-35.9158, -69.9436) (-35.9908, -69.6833) knots 0 0 0 0 1 1 1 1
  spline S162 degree 3 poles (-35.9908, -69.6833) (-36.0475, -69.4864) (-36.1068, -69.3943) (-36.2588, -69.2673) knots 0 0 0 0 1 1 1 1
  spline S163 degree 3 poles (-36.2588, -69.2673) (-36.5572, -69.0178) (-36.7051, -68.6949) (-36.7351, -68.2272) knots 0 0 0 0 1 1 1 1
  spline S164 degree 3 poles (-36.7351, -68.2272) (-36.7546, -67.9231) (-36.7839, -67.8017) (-36.8716, -67.6624) knots 0 0 0 0 1 1 1 1
  spline S165 degree 3 poles (-36.8716, -67.6624) (-37.0892, -67.3168) (-37.3841, -66.6596) (-37.3841, -66.5202) knots 0 0 0 0 1 1 1 1
  spline S166 degree 3 poles (-37.3841, -66.5202) (-37.3841, -66.4224) (-37.4554, -66.2813) (-37.616, -66.0612) knots 0 0 0 0 1 1 1 1
  spline S167 degree 3 poles (-37.616, -66.0612) (-37.9268, -65.6353) (-38.0221, -65.4065) (-38.0221, -65.0859) knots 0 0 0 0 1 1 1 1
  spline S168 degree 3 poles (-38.0221, -65.0859) (-38.0221, -64.8763) (-38.0416, -64.8058) (-38.1185, -64.7365) knots 0 0 0 0 1 1 1 1
  spline S169 degree 3 poles (-38.1185, -64.7365) (-38.2777, -64.593) (-38.4922, -64.0881) (-38.4972, -63.8448) knots 0 0 0 0 1 1 1 1
  spline S170 degree 3 poles (-38.4972, -63.8448) (-38.5012, -63.6545) (-38.5254, -63.6025) (-38.6896, -63.432) knots 0 0 0 0 1 1 1 1
  spline S171 degree 3 poles (-38.6896, -63.432) (-39.0848, -63.0217) (-39.2763, -62.5524) (-39.1944, -62.1947) knots 0 0 0 0 1 1 1 1
  spline S172 degree 3 poles (-39.1944, -62.1947) (-39.151, -62.0051) (-39.1565, -61.9799) (-39.271, -61.8438) knots 0 0 0 0 1 1 1 1
  spline S173 degree 3 poles (-39.271, -61.8438) (-39.5749, -61.4827) (-39.7064, -61.0329) (-39.6201, -60.6505) knots 0 0 0 0 1 1 1 1
  spline S174 degree 3 poles (-39.6201, -60.6505) (-39.5743, -60.4475) (-39.5791, -60.423) (-39.698, -60.259) knots 0 0 0 0 1 1 1 1
  spline S175 degree 3 poles (-39.698, -60.259) (-39.7677, -60.1627) (-39.8611, -60.0038) (-39.9055, -59.9059) knots 0 0 0 0 1 1 1 1
  spline S176 degree 3 poles (-39.9055, -59.9059) (-39.9612, -59.783) (-40.081, -59.6605) (-40.2916, -59.511) knots 0 0 0 0 1 1 1 1
  spline S177 degree 3 poles (-40.2916, -59.511) (-41.0321, -58.9854) (-43.0088, -57.5318) (-43.198, -57.3738) knots 0 0 0 0 1 1 1 1
  spline S178 degree 3 poles (-43.198, -57.3738) (-43.2684, -57.3149) (-43.4092, -57.1928) (-43.511, -57.1023) knots 0 0 0 0 1 1 1 1
  spline S179 degree 3 poles (-43.511, -57.1023) (-43.6127, -57.0118) (-43.8981, -56.7804) (-44.1451, -56.5881) knots 0 0 0 0 1 1 1 1
  line L14 (-44.1451, -56.5881) -> (-44.5942, -56.2385)
  line L15 (-44.5942, -56.2385) -> (-44.9199, -56.2631)
  spline S180 degree 3 poles (-44.9199, -56.2631) (-45.3621, -56.2965) (-48.1545, -56.3703) (-50.213, -56.403) knots 0 0 0 0 1 1 1 1
  spline S181 degree 3 poles (-50.213, -56.403) (-51.1404, -56.4178) (-52.3914, -56.4601) (-52.9929, -56.497) knots 0 0 0 0 1 1 1 1
  spline S182 degree 3 poles (-52.9929, -56.497) (-53.8407, -56.5491) (-54.9325, -56.5612) (-57.8465, -56.5509) knots 0 0 0 0 1 1 1 1
  spline S183 degree 3 poles (-57.8465, -56.5509) (-62.7312, -56.5337) (-63.9953, -56.543) (-64.6564, -56.6012) knots 0 0 0 0 1 1 1 1
  spline S184 degree 3 poles (-64.6564, -56.6012) (-65.0967, -56.64) (-65.283, -56.6361) (-65.6363, -56.5807) knots 0 0 0 0 1 1 1 1
  spline S185 degree 3 poles (-65.6363, -56.5807) (-66.1781, -56.4958) (-66.2885, -56.4524) (-66.4601, -56.257) knots 0 0 0 0 1 1 1 1
  spline S186 degree 3 poles (-66.4601, -56.257) (-66.6314, -56.0618) (-66.6367, -55.8859) (-66.4769, -55.696) knots 0 0 0 0 1 1 1 1
  spline S187 degree 3 poles (-24.967, -41.4757) (-24.9553, -41.4757) (-24.9212, -41.4295) (-24.8912, -41.3731) knots 0 0 0 0 1 1 1 1
  spline S188 degree 3 poles (-24.8912, -41.3731) (-24.8416, -41.2802) (-24.8436, -41.2764) (-24.9124, -41.3331) knots 0 0 0 0 1 1 1 1
  spline S189 degree 3 poles (-24.9124, -41.3331) (-24.9829, -41.3914) (-25.0153, -41.4757) (-24.967, -41.4757) knots 0 0 0 0 1 1 1 1
extrude "Extrusion8" cut sketch "Skizze5" against normal blind 0.4 contours S0 S1 L0 L1 S2 S3 L2 L3 S4 L4 L5 S5 L6 L7 S6 S7 S8 S9 S10 S11 S12 S13 S14 S15 S16 L8 L9 S17 S18 S19 S20 S21 S22 S23 S24 S25 S26 S27 S28 S29 S30 S31 S32 S33 S34 S35 S36 S37 S38 S39 S40 S41 S42 S43 S44 S45 S46 S47 S48 S49 S50 S51 S52 S53 S54 S55 S56 S57 S58 S59 S60 S61 S62 S63 S64 S65 S66 L10 L11 S67 S68 S69 S70 S71 S72 S73 S74 L12 L13 S75 S76 S77 S78 S79 S80 S81 S82 S83 S84 S85 S86 S87 S88 S89 S90 S91 S92 S93 S94 S95 S96 S97 S98 S99 S100 S101 S102 S103 S104 S105 S106 S107 S108 S109 S110 S111 S112 S113 S114 S115 S116 S117 S118 S119 S120 S121 S122 S123 S124 S125 S126 S127 S128 S129 S130 S131 S132 S133 S134 S135 S136 S137 S138 S139 S140 S141 S142 S143 S144 S145 S146 S147 S148 S149 S150 S151 S152 S153 S154 S155 S156 S157 S158 S159 S160 S161 S162 S163 S164 S165 S166 S167 S168 S169 S170 S171 S172 S173 S174 S175 S176 S177 S178 S179 L14 L15 S180 S181 S182 S183 S184 S185 S186
extrude "Extrusion5" [suppressed]
sketch "Skizze4" plane through (0, 0, 1) normal (0, 0, 1) x (-1, 0, 0)
  arc A0 (-27.8484, -22.7143) -> (-57.1516, -22.7143) centre (-42.5, -19.5) ccw
  arc A1 (-57.1516, -22.7143) -> (-57.1516, -86.2857) centre (-42.5, -54.5) ccw
  arc A2 (-57.1516, -86.2857) -> (-27.8484, -86.2857) centre (-42.5, -89.5) ccw
  arc A3 (-27.8484, -86.2857) -> (-27.8484, -22.7143) centre (-42.5, -54.5) ccw
  spline S0 degree 3 poles (-70.5128, -55.4557) (-70.3599, -55.2739) (-70.0727, -55.115) (-69.7047, -55.0084) knots 0 0 0 0 1 1 1 1
  spline S1 degree 3 poles (-69.7047, -55.0084) (-69.4517, -54.9352) (-68.2513, -54.8913) (-64.325, -54.8116) knots 0 0 0 0 1 1 1 1
  line L0 (-64.325, -54.8116) -> (-62.8653, -54.782)
  line L1 (-62.8653, -54.782) -> (-62.8076, -54.6426)
  spline S2 degree 3 poles (-62.8076, -54.6426) (-62.7759, -54.566) (-62.6293, -54.3841) (-62.4818, -54.2385) knots 0 0 0 0 1 1 1 1
  spline S3 degree 3 poles (-62.4818, -54.2385) (-62.2756, -54.0349) (-62.1265, -53.9419) (-61.8355, -53.8357) knots 0 0 0 0 1 1 1 1
  line L2 (-61.8355, -53.8357) -> (-61.4572, -53.6976)
  line L3 (-61.4572, -53.6976) -> (-59.1408, -53.6905)
  spline S4 degree 3 poles (-59.1408, -53.6905) (-57.8667, -53.6866) (-56.4854, -53.6981) (-56.0712, -53.716) knots 0 0 0 0 1 1 1 1
  line L4 (-56.0712, -53.716) -> (-55.318, -53.7485)
  line L5 (-55.318, -53.7485) -> (-55.1293, -53.5533)
  spline S5 degree 3 poles (-55.1293, -53.5533) (-54.751, -53.1618) (-54.6567, -53.137) (-53.5702, -53.1423) knots 0 0 0 0 1 1 1 1
  line L6 (-53.5702, -53.1423) -> (-52.607, -53.1471)
  line L7 (-52.607, -53.1471) -> (-52.8575, -53.0279)
  spline S6 degree 3 poles (-52.8575, -53.0279) (-53.3329, -52.8016) (-53.5118, -52.4679) (-53.2755, -52.2478) knots 0 0 0 0 1 1 1 1
  spline S7 degree 3 poles (-53.2755, -52.2478) (-53.1098, -52.0933) (-52.8185, -52.0302) (-52.1915, -52.0129) knots 0 0 0 0 1 1 1 1
  spline S8 degree 3 poles (-52.1915, -52.0129) (-51.8835, -52.0043) (-51.62, -51.9959) (-51.606, -51.9941) knots 0 0 0 0 1 1 1 1
  spline S9 degree 3 poles (-51.606, -51.9941) (-51.592, -51.9923) (-51.7167, -51.9151) (-51.8831, -51.8226) knots 0 0 0 0 1 1 1 1
  spline S10 degree 3 poles (-51.8831, -51.8226) (-52.2961, -51.5928) (-52.3951, -51.4486) (-52.3951, -51.0773) knots 0 0 0 0 1 1 1 1
  spline S11 degree 3 poles (-52.3951, -51.0773) (-52.3951, -50.8529) (-52.3704, -50.7532) (-52.2933, -50.6668) knots 0 0 0 0 1 1 1 1
  spline S12 degree 3 poles (-52.2933, -50.6668) (-52.1386, -50.4932) (-51.879, -50.4018) (-51.6505, -50.4404) knots 0 0 0 0 1 1 1 1
  spline S13 degree 3 poles (-51.6505, -50.4404) (-51.4235, -50.4788) (-51.4048, -50.436) (-51.577, -50.2728) knots 0 0 0 0 1 1 1 1
  spline S14 degree 3 poles (-51.577, -50.2728) (-51.6441, -50.2092) (-51.7287, -50.0411) (-51.7651, -49.8993) knots 0 0 0 0 1 1 1 1
  spline S15 degree 3 poles (-51.7651, -49.8993) (-51.8123, -49.7149) (-51.8791, -49.6028) (-51.9997, -49.5058) knots 0 0 0 0 1 1 1 1
  spline S16 degree 3 poles (-51.9997, -49.5058) (-53.1562, -48.5749) (-53.5153, -48.0897) (-53.515, -47.4582) knots 0 0 0 0 1 1 1 1
  line L8 (-53.515, -47.4582) -> (-53.515, -47.1245)
  line L9 (-53.515, -47.1245) -> (-53.9874, -46.7709)
  spline S17 degree 3 poles (-53.9874, -46.7709) (-55.0888, -45.9468) (-56.3902, -44.9397) (-56.8456, -44.5591) knots 0 0 0 0 1 1 1 1
  spline S18 degree 3 poles (-56.8456, -44.5591) (-57.0299, -44.4051) (-57.289, -44.1921) (-57.4213, -44.0858) knots 0 0 0 0 1 1 1 1
  spline S19 degree 3 poles (-57.4213, -44.0858) (-57.5536, -43.9795) (-57.6911, -43.865) (-57.7268, -43.8313) knots 0 0 0 0 1 1 1 1
  spline S20 degree 3 poles (-57.7268, -43.8313) (-57.7626, -43.7976) (-57.9636, -43.6212) (-58.1736, -43.4392) knots 0 0 0 0 1 1 1 1
  spline S21 degree 3 poles (-58.1736, -43.4392) (-58.3835, -43.2572) (-58.5668, -43.096) (-58.5808, -43.0809) knots 0 0 0 0 1 1 1 1
  spline S22 degree 3 poles (-58.5808, -43.0809) (-58.5948, -43.0657) (-58.8468, -42.8643) (-59.1408, -42.6331) knots 0 0 0 0 1 1 1 1
  spline S23 degree 3 poles (-59.1408, -42.6331) (-60.1614, -41.8307) (-60.957, -41.1966) (-61.0541, -41.1082) knots 0 0 0 0 1 1 1 1
  spline S24 degree 3 poles (-61.0541, -41.1082) (-61.1078, -41.0593) (-61.2175, -40.9684) (-61.2978, -40.9062) knots 0 0 0 0 1 1 1 1
  spline S25 degree 3 poles (-61.2978, -40.9062) (-61.555, -40.7071) (-61.946, -40.3434) (-62.8083, -39.5013) knots 0 0 0 0 1 1 1 1
  spline S26 degree 3 poles (-62.8083, -39.5013) (-63.2714, -39.049) (-63.8096, -38.5416) (-64.0042, -38.3736) knots 0 0 0 0 1 1 1 1
  spline S27 degree 3 poles (-64.0042, -38.3736) (-64.6201, -37.842) (-65.0155, -37.4652) (-65.2342, -37.2014) knots 0 0 0 0 1 1 1 1
  spline S28 degree 3 poles (-65.2342, -37.2014) (-65.7056, -36.633) (-65.8474, -36.0722) (-65.5741, -35.8572) knots 0 0 0 0 1 1 1 1
  spline S29 degree 3 poles (-65.5741, -35.8572) (-65.5003, -35.7992) (-65.39, -35.7517) (-65.329, -35.7517) knots 0 0 0 0 1 1 1 1
  spline S30 degree 3 poles (-65.329, -35.7517) (-65.06, -35.7517) (-64.4776, -36.124) (-63.5627, -36.8808) knots 0 0 0 0 1 1 1 1
  spline S31 degree 3 poles (-63.5627, -36.8808) (-62.9197, -37.4126) (-60.8771, -39.2031) (-60.4101, -39.6443) knots 0 0 0 0 1 1 1 1
  spline S32 degree 3 poles (-60.4101, -39.6443) (-59.7298, -40.287) (-58.8201, -41.0372) (-58.1545, -41.5042) knots 0 0 0 0 1 1 1 1
  spline S33 degree 3 poles (-58.1545, -41.5042) (-58.0949, -41.546) (-57.8285, -41.7476) (-57.5625, -41.9521) knots 0 0 0 0 1 1 1 1
  spline S34 degree 3 poles (-57.5625, -41.9521) (-57.2965, -42.1566) (-56.9071, -42.4539) (-56.6971, -42.6128) knots 0 0 0 0 1 1 1 1
  spline S35 degree 3 poles (-56.6971, -42.6128) (-56.4871, -42.7717) (-56.3038, -42.9149) (-56.2898, -42.931) knots 0 0 0 0 1 1 1 1
  spline S36 degree 3 poles (-56.2898, -42.931) (-56.1978, -43.0367) (-55.4294, -43.5794) (-54.5334, -44.1715) knots 0 0 0 0 1 1 1 1
  spline S37 degree 3 poles (-54.5334, -44.1715) (-54.2814, -44.338) (-53.8489, -44.648) (-53.5724, -44.8604) knots 0 0 0 0 1 1 1 1
  spline S38 degree 3 poles (-53.5724, -44.8604) (-53.2959, -45.0727) (-52.7899, -45.4527) (-52.4479, -45.7047) knots 0 0 0 0 1 1 1 1
  spline S39 degree 3 poles (-52.4479, -45.7047) (-52.106, -45.9567) (-51.7143, -46.2545) (-51.5776, -46.3665) knots 0 0 0 0 1 1 1 1
  spline S40 degree 3 poles (-51.5776, -46.3665) (-51.4408, -46.4785) (-51.2825, -46.6079) (-51.2257, -46.6541) knots 0 0 0 0 1 1 1 1
  spline S41 degree 3 poles (-51.2257, -46.6541) (-50.9212, -46.9016) (-50.5822, -47.1969) (-50.3333, -47.4313) knots 0 0 0 0 1 1 1 1
  spline S42 degree 3 poles (-50.3333, -47.4313) (-49.7991, -47.9343) (-49.082, -48.5194) (-48.3007, -49.0895) knots 0 0 0 0 1 1 1 1
  spline S43 degree 3 poles (-48.3007, -49.0895) (-47.8688, -49.4047) (-47.4586, -49.7153) (-47.3892, -49.7796) knots 0 0 0 0 1 1 1 1
  spline S44 degree 3 poles (-47.3892, -49.7796) (-47.3198, -49.844) (-47.1374, -49.9447) (-46.9839, -50.0035) knots 0 0 0 0 1 1 1 1
  spline S45 degree 3 poles (-46.9839, -50.0035) (-46.8303, -50.0622) (-46.5587, -50.2123) (-46.3802, -50.3371) knots 0 0 0 0 1 1 1 1
  spline S46 degree 3 poles (-46.3802, -50.3371) (-46.2018, -50.4618) (-45.9587, -50.6182) (-45.8399, -50.6846) knots 0 0 0 0 1 1 1 1
  spline S47 degree 3 poles (-45.8399, -50.6846) (-45.7212, -50.751) (-45.4179, -50.9212) (-45.1658, -51.0627) knots 0 0 0 0 1 1 1 1
  spline S48 degree 3 poles (-45.1658, -51.0627) (-44.5263, -51.4219) (-44.285, -51.5252) (-43.6131, -51.7274) knots 0 0 0 0 1 1 1 1
  spline S49 degree 3 poles (-43.6131, -51.7274) (-43.5151, -51.7569) (-43.2516, -51.8146) (-43.0276, -51.8555) knots 0 0 0 0 1 1 1 1
  spline S50 degree 3 poles (-43.0276, -51.8555) (-41.6327, -52.1108) (-41.0767, -52.1689) (-40.9684, -52.0709) knots 0 0 0 0 1 1 1 1
  spline S51 degree 3 poles (-40.9684, -52.0709) (-40.9248, -52.0314) (-40.8262, -51.9753) (-40.7493, -51.946) knots 0 0 0 0 1 1 1 1
  spline S52 degree 3 poles (-40.7493, -51.946) (-40.6309, -51.901) (-40.6093, -51.8632) (-40.6089, -51.7006) knots 0 0 0 0 1 1 1 1
  spline S53 degree 3 poles (-40.6089, -51.7006) (-40.6083, -51.4664) (-40.3825, -51.0534) (-40.1372, -50.8381) knots 0 0 0 0 1 1 1 1
  spline S54 degree 3 poles (-40.1372, -50.8381) (-40.0411, -50.7537) (-39.7877, -50.5722) (-39.574, -50.4347) knots 0 0 0 0 1 1 1 1
  spline S55 degree 3 poles (-39.574, -50.4347) (-39.2319, -50.2146) (-39.1854, -50.1665) (-39.1847, -50.0313) knots 0 0 0 0 1 1 1 1
  spline S56 degree 3 poles (-39.1847, -50.0313) (-39.1835, -49.8048) (-39.0089, -49.5109) (-38.67, -49.1652) knots 0 0 0 0 1 1 1 1
  spline S57 degree 3 poles (-38.67, -49.1652) (-38.4386, -48.929) (-38.3693, -48.8233) (-38.3693, -48.7063) knots 0 0 0 0 1 1 1 1
  spline S58 degree 3 poles (-38.3693, -48.7063) (-38.3693, -48.417) (-38.1267, -48.0823) (-37.2826, -47.2065) knots 0 0 0 0 1 1 1 1
  spline S59 degree 3 poles (-37.2826, -47.2065) (-37.1426, -47.0614) (-37.0493, -46.911) (-37.0277, -46.796) knots 0 0 0 0 1 1 1 1
  spline S60 degree 3 poles (-37.0277, -46.796) (-36.9882, -46.5854) (-36.8058, -46.3959) (-36.3345, -46.0759) knots 0 0 0 0 1 1 1 1
  spline S61 degree 3 poles (-36.3345, -46.0759) (-36.0776, -45.9016) (-35.9978, -45.8167) (-35.9721, -45.6907) knots 0 0 0 0 1 1 1 1
  spline S62 degree 3 poles (-35.9721, -45.6907) (-35.9341, -45.5053) (-35.8028, -45.2888) (-35.6495, -45.1589) knots 0 0 0 0 1 1 1 1
  spline S63 degree 3 poles (-35.6495, -45.1589) (-35.4716, -45.0083) (-34.9499, -44.7628) (-34.8076, -44.7628) knots 0 0 0 0 1 1 1 1
  spline S64 degree 3 poles (-34.8076, -44.7628) (-34.6243, -44.7628) (-34.551, -44.675) (-34.551, -44.455) knots 0 0 0 0 1 1 1 1
  spline S65 degree 3 poles (-34.551, -44.455) (-34.551, -44.204) (-34.4304, -43.9703) (-34.1512, -43.6806) knots 0 0 0 0 1 1 1 1
  spline S66 degree 3 poles (-34.1512, -43.6806) (-33.9698, -43.4924) (-33.8254, -43.4035) (-33.5037, -43.2821) knots 0 0 0 0 1 1 1 1
  line L10 (-33.5037, -43.2821) -> (-33.0896, -43.1258)
  line L11 (-33.0896, -43.1258) -> (-32.9422, -42.8175)
  spline S67 degree 3 poles (-32.9422, -42.8175) (-32.8588, -42.6429) (-32.7032, -42.4286) (-32.5834, -42.3231) knots 0 0 0 0 1 1 1 1
  spline S68 degree 3 poles (-32.5834, -42.3231) (-32.3307, -42.1007) (-31.8601, -41.8609) (-31.6762, -41.8609) knots 0 0 0 0 1 1 1 1
  spline S69 degree 3 poles (-31.6762, -41.8609) (-31.6036, -41.8609) (-31.5356, -41.8323) (-31.5251, -41.7973) knots 0 0 0 0 1 1 1 1
  spline S70 degree 3 poles (-31.5251, -41.7973) (-31.3819, -41.3186) (-31.3166, -41.1568) (-31.21, -41.017) knots 0 0 0 0 1 1 1 1
  spline S71 degree 3 poles (-31.21, -41.017) (-31.0589, -40.819) (-30.989, -40.7846) (-30.6567, -40.7454) knots 0 0 0 0 1 1 1 1
  spline S72 degree 3 poles (-30.6567, -40.7454) (-30.4372, -40.7195) (-30.399, -40.6981) (-30.3767, -40.5882) knots 0 0 0 0 1 1 1 1
  spline S73 degree 3 poles (-30.3767, -40.5882) (-30.3625, -40.5182) (-30.2868, -40.3464) (-30.2085, -40.2063) knots 0 0 0 0 1 1 1 1
  spline S74 degree 3 poles (-30.2085, -40.2063) (-29.947, -39.7389) (-29.389, -39.4803) (-28.8307, -39.5677) knots 0 0 0 0 1 1 1 1
  line L12 (-28.8307, -39.5677) -> (-28.5833, -39.6064)
  line L13 (-28.5833, -39.6064) -> (-28.507, -39.4227)
  spline S75 degree 3 poles (-28.507, -39.4227) (-28.1036, -38.4508) (-27.7892, -38.1445) (-27.195, -38.1445) knots 0 0 0 0 1 1 1 1
  spline S76 degree 3 poles (-27.195, -38.1445) (-26.9909, -38.1445) (-26.9559, -38.1277) (-26.9019, -38.0045) knots 0 0 0 0 1 1 1 1
  spline S77 degree 3 poles (-26.9019, -38.0045) (-26.772, -37.7076) (-26.4075, -37.1856) (-26.2535, -37.076) knots 0 0 0 0 1 1 1 1
  spline S78 degree 3 poles (-26.2535, -37.076) (-26.1154, -36.9776) (-25.9897, -36.9426) (-25.7156, -36.9259) knots 0 0 0 0 1 1 1 1
  spline S79 degree 3 poles (-25.7156, -36.9259) (-25.6862, -36.9241) (-25.6323, -36.8367) (-25.5958, -36.7317) knots 0 0 0 0 1 1 1 1
  spline S80 degree 3 poles (-25.5958, -36.7317) (-25.3925, -36.1469) (-24.9937, -35.4483) (-24.7735, -35.2915) knots 0 0 0 0 1 1 1 1
  spline S81 degree 3 poles (-24.7735, -35.2915) (-24.5827, -35.1557) (-24.454, -35.1952) (-24.346, -35.4226) knots 0 0 0 0 1 1 1 1
  spline S82 degree 3 poles (-24.346, -35.4226) (-24.3, -35.5196) (-24.2462, -35.5989) (-24.2266, -35.5988) knots 0 0 0 0 1 1 1 1
  spline S83 degree 3 poles (-24.2266, -35.5988) (-24.2069, -35.5987) (-24.1476, -35.4935) (-24.0947, -35.3651) knots 0 0 0 0 1 1 1 1
  spline S84 degree 3 poles (-24.0947, -35.3651) (-23.7392, -34.5007) (-22.6012, -33.4049) (-22.4549, -33.7862) knots 0 0 0 0 1 1 1 1
  spline S85 degree 3 poles (-22.4549, -33.7862) (-22.431, -33.8483) (-22.6074, -34.4109) (-22.7917, -34.8608) knots 0 0 0 0 1 1 1 1
  spline S86 degree 3 poles (-22.7917, -34.8608) (-22.8639, -35.0368) (-22.8843, -35.0902) (-23.0638, -35.5735) knots 0 0 0 0 1 1 1 1
  spline S87 degree 3 poles (-23.0638, -35.5735) (-23.2012, -35.9433) (-23.2806, -36.2608) (-23.2358, -36.2608) knots 0 0 0 0 1 1 1 1
  spline S88 degree 3 poles (-23.2358, -36.2608) (-23.2215, -36.2608) (-23.0656, -36.0603) (-22.8893, -35.8153) knots 0 0 0 0 1 1 1 1
  spline S89 degree 3 poles (-22.8893, -35.8153) (-22.5065, -35.2832) (-21.4698, -34.033) (-21.1561, -33.7249) knots 0 0 0 0 1 1 1 1
  spline S90 degree 3 poles (-21.1561, -33.7249) (-20.7571, -33.3331) (-20.2452, -33.0425) (-20.2452, -33.2077) knots 0 0 0 0 1 1 1 1
  spline S91 degree 3 poles (-20.2452, -33.2077) (-20.2452, -33.2366) (-20.4686, -33.5203) (-20.7416, -33.8382) knots 0 0 0 0 1 1 1 1
  spline S92 degree 3 poles (-20.7416, -33.8382) (-21.3238, -34.5161) (-21.4905, -34.7265) (-21.6924, -35.0381) knots 0 0 0 0 1 1 1 1
  spline S93 degree 3 poles (-21.6924, -35.0381) (-21.9463, -35.4299) (-22.2331, -35.9699) (-22.2033, -35.9997) knots 0 0 0 0 1 1 1 1
  spline S94 degree 3 poles (-22.2033, -35.9997) (-22.1876, -36.0154) (-21.7922, -35.6412) (-21.3246, -35.1681) knots 0 0 0 0 1 1 1 1
  spline S95 degree 3 poles (-21.3246, -35.1681) (-20.6638, -34.4998) (-20.3569, -34.2307) (-19.9476, -33.9608) knots 0 0 0 0 1 1 1 1
  spline S96 degree 3 poles (-19.9476, -33.9608) (-19.652, -33.7658) (-19.3654, -33.6135) (-19.2943, -33.6135) knots 0 0 0 0 1 1 1 1
  spline S97 degree 3 poles (-19.2943, -33.6135) (-19.1019, -33.6135) (-19.1715, -33.7141) (-19.5299, -33.9542) knots 0 0 0 0 1 1 1 1
  spline S98 degree 3 poles (-19.5299, -33.9542) (-19.9191, -34.215) (-20.3372, -34.5746) (-20.88, -35.1154) knots 0 0 0 0 1 1 1 1
  spline S99 degree 3 poles (-20.88, -35.1154) (-21.6328, -35.8655) (-22.0277, -36.3799) (-22.6688, -37.4461) knots 0 0 0 0 1 1 1 1
  spline S100 degree 3 poles (-22.6688, -37.4461) (-23.0466, -38.0745) (-23.0673, -38.1768) (-22.7581, -37.888) knots 0 0 0 0 1 1 1 1
  spline S101 degree 3 poles (-22.7581, -37.888) (-22.5056, -37.6522) (-22.3308, -37.5071) (-21.5689, -36.9008) knots 0 0 0 0 1 1 1 1
  spline S102 degree 3 poles (-21.5689, -36.9008) (-21.3309, -36.7114) (-20.9872, -36.4154) (-20.8052, -36.2429) knots 0 0 0 0 1 1 1 1
  spline S103 degree 3 poles (-20.8052, -36.2429) (-20.1416, -35.614) (-19.6857, -35.2364) (-19.1692, -34.8877) knots 0 0 0 0 1 1 1 1
  spline S104 degree 3 poles (-19.1692, -34.8877) (-18.879, -34.6919) (-18.5302, -34.451) (-18.3942, -34.3525) knots 0 0 0 0 1 1 1 1
  spline S105 degree 3 poles (-18.3942, -34.3525) (-18.1465, -34.1732) (-17.9875, -34.1293) (-17.9291, -34.224) knots 0 0 0 0 1 1 1 1
  spline S106 degree 3 poles (-17.9291, -34.224) (-17.8923, -34.2834) (-18.0033, -34.3896) (-18.5683, -34.8353) knots 0 0 0 0 1 1 1 1
  spline S107 degree 3 poles (-18.5683, -34.8353) (-19.6967, -35.7254) (-20.4652, -36.4138) (-21.4569, -37.4229) knots 0 0 0 0 1 1 1 1
  spline S108 degree 3 poles (-21.4569, -37.4229) (-22.0534, -38.0298) (-22.6376, -38.6594) (-22.7551, -38.822) knots 0 0 0 0 1 1 1 1
  spline S109 degree 3 poles (-22.7551, -38.822) (-22.8727, -38.9846) (-23.0627, -39.2405) (-23.1774, -39.3907) knots 0 0 0 0 1 1 1 1
  spline S110 degree 3 poles (-23.1774, -39.3907) (-23.6835, -40.0535) (-24.595, -41.4931) (-24.9672, -42.2173) knots 0 0 0 0 1 1 1 1
  spline S111 degree 3 poles (-24.9672, -42.2173) (-25.4976, -43.2495) (-25.6646, -43.5368) (-26.163, -44.2748) knots 0 0 0 0 1 1 1 1
  spline S112 degree 3 poles (-26.163, -44.2748) (-27.1088, -45.6751) (-27.78, -46.7144) (-27.78, -46.7788) knots 0 0 0 0 1 1 1 1
  spline S113 degree 3 poles (-27.78, -46.7788) (-27.78, -46.7912) (-27.8337, -46.8867) (-27.8995, -46.9912) knots 0 0 0 0 1 1 1 1
  spline S114 degree 3 poles (-27.8995, -46.9912) (-27.9652, -47.0956) (-28.0996, -47.33) (-28.198, -47.512) knots 0 0 0 0 1 1 1 1
  spline S115 degree 3 poles (-28.198, -47.512) (-28.2965, -47.694) (-28.4299, -47.9345) (-28.4946, -48.0466) knots 0 0 0 0 1 1 1 1
  spline S116 degree 3 poles (-28.4946, -48.0466) (-28.5593, -48.1586) (-28.6715, -48.3533) (-28.7438, -48.4793) knots 0 0 0 0 1 1 1 1
  spline S117 degree 3 poles (-28.7438, -48.4793) (-28.8162, -48.6053) (-28.9554, -48.8217) (-29.0532, -48.9602) knots 0 0 0 0 1 1 1 1
  spline S118 degree 3 poles (-29.0532, -48.9602) (-29.3667, -49.4044) (-30.889, -51.293) (-31.8475, -52.4268) knots 0 0 0 0 1 1 1 1
  spline S119 degree 3 poles (-31.8475, -52.4268) (-32.0392, -52.6536) (-32.9064, -53.8189) (-33.1153, -54.1303) knots 0 0 0 0 1 1 1 1
  spline S120 degree 3 poles (-33.1153, -54.1303) (-33.6296, -54.8971) (-33.6882, -55.0195) (-33.6805, -55.3097) knots 0 0 0 0 1 1 1 1
  spline S121 degree 3 poles (-33.6805, -55.3097) (-33.6671, -55.8139) (-33.4355, -56.192) (-32.8539, -56.6587) knots 0 0 0 0 1 1 1 1
  spline S122 degree 3 poles (-32.8539, -56.6587) (-31.8565, -57.4592) (-31.3983, -58.0944) (-31.1596, -59.0075) knots 0 0 0 0 1 1 1 1
  spline S123 degree 3 poles (-31.1596, -59.0075) (-31.0738, -59.336) (-31.0653, -60.4309) (-31.1471, -60.6318) knots 0 0 0 0 1 1 1 1
  spline S124 degree 3 poles (-31.1471, -60.6318) (-31.5226, -61.554) (-31.9033, -62.0615) (-32.4269, -62.3379) knots 0 0 0 0 1 1 1 1
  spline S125 degree 3 poles (-32.4269, -62.3379) (-32.7324, -62.4991) (-33.4553, -62.4983) (-33.7842, -62.3363) knots 0 0 0 0 1 1 1 1
  spline S126 degree 3 poles (-33.7842, -62.3363) (-34.2557, -62.1042) (-34.3216, -62.1932) (-34.1268, -62.7988) knots 0 0 0 0 1 1 1 1